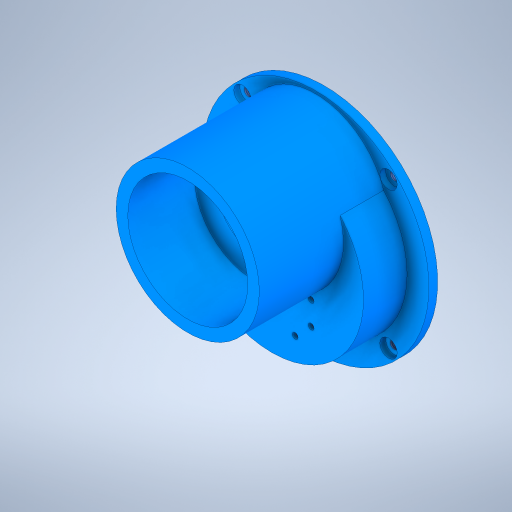
# Autodesk Inventor part: B-03
Saved by Autodesk Inventor 2024.3 (Build 283343000, 343)
## iProperties
Created: 2022-03-24
Part Number: B-03
Material: PETG
Document SubType Name: Modeling
Designer: Alcatraz
Density: 1.27 g/cm^3
Appearance: Genérico
Author: Alcatraz
Autodesk Inventor part; units mm, degrees
ref_plane "YZ Plane" through (0, 0, 0) normal (1, 0, 0) x (0, 1, 0)
ref_plane "XZ Plane" through (0, 0, 0) normal (0, 1, 0) x (-1, 0, 0)
ref_plane "XY Plane" through (0, 0, 0) normal (0, 0, 1) x (1, 0, 0)
sketch "Boceto1" plane through (0, 0, 0) normal (0, 0, 1) x (1, 0, 0)
  circle A0 centre (0, 0) radius 39
  circle A1 centre (0, 0) radius 29
  circle A2 centre (0, 0) radius 31.5
  dimension "DiametroExterior" = 78
  dimension "DiametroCaja" = 58
  dimension "d2" = 63
  constraints: 3 centre point, 3 coincident
  measures "DiametroExterior" diameter of A0
  measures "DiametroCaja" diameter of A1
  measures "d2" diameter of A2
extrude "Extrusión1" add sketch "Boceto1" along normal blind 18 contours A2
sketch "Boceto2" plane through (0, 0, 18) normal (0, 0, 1) x (1, 0, 0)
  circle A0 centre (0, 0) radius 39
  circle A1 centre (0, 0) radius 31
  dimension "d5" = 78
  dimension "d6" = 62
  constraints: 2 centre point, 2 coincident
  measures "d5" diameter of A0
  measures "d6" diameter of A1
extrude "Extrusión2" add sketch "Boceto2" against normal blind 3
sketch "Boceto3" plane through (0, 0, 0) normal (0, 0, -1) x (-1, 0, 0)
  circle A0 centre (0, 0) radius 29
  dimension "d9" = 58
  constraints: 1 centre point, 1 coincident
  measures "d9" diameter of A0
extrude "Extrusión3" add sketch "Boceto3" against normal blind 6
sketch "Boceto5" plane through (0, 0, 15) normal (0, 0, -1) x (-1, 0, 0)
  line L0 (0, 0) -> (33, 0) construction
  line L1 (0, 0) -> (33.75, 0) construction
  circle A0 centre (0, 0) radius 39
  circle A1 centre (0, 0) radius 31.5
  circle A2 centre (25.1022, 25.1024) radius 2
  circle A3 centre (25.1024, -25.1022) radius 2
  circle A4 centre (-25.1022, -25.1024) radius 2
  circle A5 centre (-25.1024, 25.1022) radius 2
  point P0 (23.8649, 23.8649)
  dimension "d14" = 33.75
  dimension "d81" = 78
  dimension "d82" = 63
  dimension "d83" = 4
  dimension "d84" = 2
  dimension "d85" = 1.5
  dimension "d86" = 360
  constraints: 6 centre point, 4 coincident, 4 end point, 2 horizontal, 11 other
  measures "d14" distance of L0.start point (23.865, 23.865)
  measures "d81" diameter of A0
  measures "d82" diameter of A1
  measures "d83" diameter of A2
sketch "Boceto6" plane through (0, 0, 6) normal (0, 0, 1) x (1, 0, 0)
  line L0 (-16, -25) -> (16, -25)
  line L1 (16, -25) -> (16, 25)
  line L2 (16, 25) -> (-16, 25)
  line L3 (-16, 25) -> (-16, -25)
  line L4 (-16, -25) -> (16, 25) construction
  line L5 (16, -25) -> (-16, 25) construction
  circle A0 centre (0, 13.5) radius 12.5
  circle A1 centre (-8, -22.5) radius 1.1
  circle A2 centre (8, -22.5) radius 1.1
  circle A3 centre (13.5, -17) radius 1.1
  circle A4 centre (-13.5, -17) radius 1.1
  circle A5 centre (-13.5, -9) radius 1.1
  circle A6 centre (-13.5, -1) radius 1.1
  circle A7 centre (-13.5, 7) radius 1.1
  circle A8 centre (13.5, 7) radius 1.1
  circle A9 centre (13.5, -1) radius 1.1
  circle A10 centre (13.5, -9) radius 1.1
  line L6 (0, -25) -> (0, -19)
  line L7 (0, -19) -> (-8.307, -19)
  line L8 (0, -19) -> (8.307, -19)
  line L9 (-11.657, -15.65) -> (-11.657, 6.356)
  line L10 (11.657, -15.65) -> (11.657, 6.356)
  line L11 (10.857, 7.156) -> (9.815, 7.156)
  line L12 (-10.857, 7.156) -> (-9.815, 7.156)
  arc A11 (-9.015, 6.356) -> (9.015, 6.356) centre (0, 13.002) ccw
  arc A12 (9.815, 7.156) -> (9.015, 6.356) centre (9.815, 6.356) ccw
  arc A13 (11.657, 6.356) -> (10.857, 7.156) centre (10.857, 6.356) ccw
  arc A14 (-9.015, 6.356) -> (-9.815, 7.156) centre (-9.815, 6.356) ccw
  arc A15 (-10.857, 7.156) -> (-11.657, 6.356) centre (-10.857, 6.356) ccw
  arc A16 (10.857, -16.45) -> (11.657, -15.65) centre (10.857, -15.65) ccw
  arc A17 (10.857, -16.45) -> (9.107, -18.2) centre (10.857, -18.2) ccw
  arc A18 (8.307, -19) -> (9.107, -18.2) centre (8.307, -18.2) ccw
  arc A19 (-9.107, -18.2) -> (-8.307, -19) centre (-8.307, -18.2) ccw
  arc A20 (-9.107, -18.2) -> (-10.857, -16.45) centre (-10.857, -18.2) ccw
  arc A21 (-11.657, -15.65) -> (-10.857, -16.45) centre (-10.857, -15.65) ccw
  point P0 (0, 0)
  point P1 (0, 0)
  point P2 (10.7705, 7.156)
  point P3 (-10.7705, 7.156)
  point P4 (4.899, 25)
  point P5 (-4.899, 25)
  dimension "d27" = 32
  dimension "d28" = 50
  dimension "d29" = 25
  dimension "d30" = 11.5
  dimension "d31" = 2.2
  dimension "d32" = 2.2
  dimension "d33" = 2.2
  dimension "d34" = 2.2
  dimension "d35" = 2.2
  dimension "d36" = 2.2
  dimension "d37" = 2.2
  dimension "d38" = 2.2
  dimension "d39" = 2.2
  dimension "d40" = 2.2
  dimension "d41" = 27
  dimension "d42" = 16
  dimension "d43" = 36
  dimension "d44" = 30.5
  dimension "d45" = 6.5
  dimension "d46" = 8
  dimension "d47" = 8
  dimension "d48" = 8
  dimension "d49" = 8
  dimension "d50" = 8
  dimension "d51" = 8
  dimension "d52" = 6
  dimension "d53" = 8.307
  dimension "d54" = 22.006
  dimension "d55" = 1.042
  dimension "d56" = 1.042
  dimension "d57" = 11.2
  dimension "d58" = 0.8
  dimension "d59" = 0.8
  dimension "d60" = 0.8
  dimension "d61" = 0.8
  dimension "d62" = 1.75
  dimension "d63" = 0.8
  dimension "d64" = 1.75
  dimension "d65" = 0.8
  constraints: 26 end point, 23 point on circle, 22 centre point, 5 horizontal, 3 midpoint, 3 tangent, 3 vertical, 2 parallel, 1 perpendicular
  measures "d27" distance of L3.start L2.start
  measures "d28" distance of L2.start L5.start
  measures "d29" diameter of A0
  measures "d30" distance from line of L2 A0.centre
  measures "d31" diameter of A1
  measures "d32" diameter of A2
  measures "d33" diameter of A3
  measures "d34" diameter of A4
  measures "d35" diameter of A5
  measures "d36" diameter of A6
  measures "d37" diameter of A7
  measures "d38" diameter of A8
  measures "d39" diameter of A9
  measures "d40" diameter of A10
  measures "d41" distance of A3.centre A4.centre
  measures "d42" distance of A2.centre A1.centre
  measures "d43" vertical distance of A1.centre A0.centre
  measures "d44" vertical distance of A4.centre A0.centre
  measures "d45" vertical distance of A7.centre A0.centre
  measures "d46" distance of A9.centre A8.centre
  measures "d47" distance of A10.centre A9.centre
  measures "d48" distance of A3.centre A10.centre
  measures "d49" distance of A5.centre A4.centre
  measures "d50" distance of A5.centre A6.centre
  measures "d51" distance of A7.centre A6.centre
  measures "d52" distance of L6.start L8.start
  measures "d53" distance of L8.start L7.end
  measures "d54" distance of L9.start L9.end
  measures "d55" distance of L11.start L11.end
  measures "d56" distance of L12.start L12.end
  measures "d57" radius of A11
  measures "d58" radius of A12
  measures "d59" radius of A13
  measures "d60" radius of A14
  measures "d61" radius of A16
  measures "d62" radius of A17
  measures "d63" radius of A18
  measures "d64" radius of A20
  measures "d65" radius of A21
extrude "Extrusión4" cut sketch "Boceto6" against normal blind 3 contours L7 A19 A20 A21 L9 A15 L12 A0 L11 A13 L10 A16 A17 A18 L8
hole "Agujero2" at (13.5, -17, 6) at (13.5, -9, 6) at (8, -22.5, 6) at (-8, -22.5, 6) at (-13.5, -9, 6) at (-13.5, -17, 6) direction (0, 0, -1) diameter 2.013 depth 7.6 thread size "M2.5x0.45" class "6H" standard "ISO Metric profile"
extrude "Extrusión6" cut sketch "Boceto6" against normal blind 6 contours A0 L2 | L2 A0 L11 A12 A11 A14 L12 | L12 A14 A11 A12 L11 A0
hole "Agujero3" at (-25.1022, 25.1024, 15) at (25.1024, 25.1022, 15) at (25.1022, -25.1024, 15) at (-25.1024, -25.1022, 15) direction (0, 0, 1) diameter 2.85 depth 10.4 counterbore diameter 6 counterbore depth 2 thread size "M3.5x0.6" class "6H" standard "ISO Metric profile"
sketch "Boceto7" plane through (0, 0, 0) normal (0, 0, -1) x (-1, 0, 0)
  arc A0 (-10.7705, 7.156) -> (10.7705, 7.156) centre (0, 13.5) ccw projected
  line L0 (0, 26) -> (0, 13.5)
  circle A1 centre (0, 13.5) radius 20.6175
  circle A2 centre (0, 13.5) radius 24.6175
  point P0 (0, 0)
  dimension "DiametroRodamiento" = 41.235
  dimension "d97" = 49.235
  constraints: 2 centre point, 2 coincident, 2 end point, 1 vertical
  measures "DiametroRodamiento" diameter of A1
  measures "d97" diameter of A2
extrude "Extrusión7" add sketch "Boceto7" along normal blind 28.934
sketch "Boceto8" plane through (0, 0, 0) normal (0, 0, -1) x (-1, 0, 0)
  circle A0 centre (0, 0) radius 31.5 projected
  circle A1 centre (0, 0) radius 31.5
  circle A2 centre (0, 13.5) radius 24.6175
  circle A3 centre (0, 13.5) radius 20.6175
  point P0 (23.4296, 21.0548)
  point P1 (-23.4296, 21.0548)
  constraints: 3 centre point, 3 coincident
extrude "Extrusión8" add sketch "Boceto8" against normal blind 15 contours A0 A3 A2 | A0 A3 picked at (0.7908, 36.6312) picked at (3.3504, 32.0101)
sketch "Boceto9" plane through (0, 13.5, 0) normal (0, 0, -1) x (-1, 0, 0)
  circle A0 centre (0, 0) radius 12.5
  circle A1 centre (0, 0) radius 20.6175
  point P0 (0, -13.5)
  constraints: 2 centre point, 1 coincident
extrude "Extrusión9" add sketch "Boceto9" along normal blind 6
equation "\"d5\" = DiametroExterior"
equation "\"d9\" = DiametroCaja"
equation "\"d83\" = d87"
equation "\"d31\" = d37"
equation "\"d32\" = d37"
equation "\"d33\" = d37"
equation "\"d35\" = d37"
equation "\"d36\" = d37"
equation "\"d38\" = d37"
equation "\"d39\" = d37"
equation "\"d40\" = d37"
equation "\"d47\" = d46"
equation "\"d48\" = d46"
equation "\"d49\" = d46"
equation "\"d50\" = d46"
equation "\"d51\" = d46"
equation "\"d87\" = 4"
